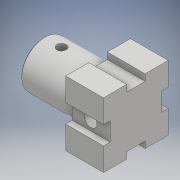
# Autodesk Inventor part: Деталь5
Saved by Autodesk Inventor 2018 (Build 220112000, 112)
## iProperties
Created: 2018-05-16
Part Number: Деталь5
Material: Типовые
Document SubType Name: Modeling
Designer: user
Density: 1 g/cm^3
Appearance: По умолчанию
Author: user
Autodesk Inventor part; units mm, degrees
ref_plane "YZ Plane" through (0, 0, 0) normal (1, 0, 0) x (0, 1, 0)
ref_plane "XZ Plane" through (0, 0, 0) normal (0, 1, 0) x (-1, 0, 0)
ref_plane "XY Plane" through (0, 0, 0) normal (0, 0, 1) x (1, 0, 0)
sketch "Эскиз1" plane through (0, 0, 0) normal (0, 0, 1) x (1, 0, 0)
  line L0 (-12.25, -21) -> (12.25, -21)
  line L1 (12.25, -21) -> (12.25, 21)
  line L2 (12.25, 21) -> (-12.25, 21)
  line L3 (-12.25, 21) -> (-12.25, -21)
  line L4 (-12.25, -21) -> (12.25, 21) construction
  line L5 (12.25, -21) -> (-12.25, 21) construction
  point P0 (0, 0)
  dimension "d0" = 24.5
  dimension "d1" = 42
  constraints: 12 end point, 2 midpoint, 2 parallel, 1 horizontal, 1 perpendicular
  measures "d0" distance of L2.end L1.end
  measures "d1" distance of L1.end L0.end
extrude "Выдавливание1" add sketch "Эскиз1" along normal mid plane 42
sketch "Эскиз2" plane through (-12.25, -21, 21) normal (-1, 0, 0) x (0, 0, 1)
  circle A0 centre (-21, 21) radius 15
  dimension "d4" = 30
  constraints: 1 centre point, 1 coincident
  measures "d4" diameter of A0
extrude "Выдавливание2" add sketch "Эскиз2" along normal blind 35
sketch "Эскиз3" plane through (-47.25, 0, 0) normal (-1, 0, 0) x (0, 0, 1)
  circle A0 centre (0, 0) radius 15 projected
  line L0 (-10, -11.1803) -> (-10, 11.1803)
  dimension "d7" = 25
  constraints: 2 end point, 2 point on circle, 1 vertical
extrude "Выдавливание3" cut sketch "Эскиз3" against normal blind 25 contours L0 A0 picked at (-11.6306, -0.5993)
chamfer "Фаска1" distance 0.5 angle 45 2 edges at (-47.25, -13.6931, 6.1237) (-47.25, 13.6931, 6.1237)
sketch "Эскиз4" plane through (-12.25, 21, 21) normal (0, 1, 0) x (1, 0, 0)
  line L0 (24.5, 42) -> (24.5, 0) projected
  line L1 (0, 15) -> (24.5, 15)
  line L2 (24.5, 15) -> (24.5, 27)
  line L3 (24.5, 27) -> (0, 27)
  line L4 (0, 27) -> (0, 15)
  line L5 (0, 15) -> (24.5, 27) construction
  line L6 (24.5, 15) -> (0, 27) construction
  point P0 (12.25, 21)
  dimension "d13" = 12
  constraints: 12 end point, 2 midpoint, 2 parallel, 1 horizontal, 1 perpendicular, 1 point on line
  measures "d13" distance of L2.end L1.end
extrude "Выдавливание4" cut sketch "Эскиз4" against normal blind 4.25
sketch "Эскиз5" plane through (-12.25, -21, 21) normal (0, -1, 0) x (1, 0, 0)
  line L0 (24.5, -42) -> (24.5, 0) projected
  line L1 (0, -15) -> (24.5, -15)
  line L2 (24.5, -15) -> (24.5, -27)
  line L3 (24.5, -27) -> (0, -27)
  line L4 (0, -27) -> (0, -15)
  line L5 (0, -15) -> (24.5, -27) construction
  line L6 (24.5, -15) -> (0, -27) construction
  point P0 (12.25, -21)
  dimension "d16" = 12
  constraints: 12 end point, 2 midpoint, 2 parallel, 1 horizontal, 1 perpendicular, 1 point on line
  measures "d16" distance of L1.end L2.end
extrude "Выдавливание5" cut sketch "Эскиз5" against normal blind 4.25
sketch "Эскиз6" plane through (0, 0, -21) normal (0, 0, -1) x (-1, 0, 0)
  line L0 (-12.25, -21) -> (-12.25, 21) projected
  line L1 (12.25, 6) -> (-12.25, 6)
  line L2 (-12.25, 6) -> (-12.25, -6)
  line L3 (-12.25, -6) -> (12.25, -6)
  line L4 (12.25, -6) -> (12.25, 6)
  line L5 (12.25, 6) -> (-12.25, -6) construction
  line L6 (-12.25, 6) -> (12.25, -6) construction
  point P0 (0, 0)
  dimension "d19" = 12
  constraints: 12 end point, 2 midpoint, 2 parallel, 1 horizontal, 1 perpendicular, 1 point on line
  measures "d19" distance of L2.end L1.end
extrude "Выдавливание6" cut sketch "Эскиз6" against normal blind 4.25
sketch "Эскиз7" plane through (0, 0, 21) normal (0, 0, 1) x (1, 0, 0)
  line L0 (-12.25, 6) -> (-12.25, -6) projected
  line L1 (12.25, 6) -> (-12.25, 6)
  line L2 (-12.25, 6) -> (-12.25, -6)
  line L3 (-12.25, -6) -> (12.25, -6)
  line L4 (12.25, -6) -> (12.25, 6)
  line L5 (12.25, 6) -> (-12.25, -6) construction
  line L6 (-12.25, 6) -> (12.25, -6) construction
  point P0 (0, 0)
  dimension "d22" = 12
  constraints: 12 end point, 2 midpoint, 2 parallel, 1 horizontal, 1 perpendicular
  measures "d22" distance of L0.end L1.end
extrude "Выдавливание7" cut sketch "Эскиз7" against normal blind 4.25
sketch "Эскиз8" plane through (-22.25, -11.1803, -10) normal (0, 0, -1) x (-1, 0, 0)
  line L0 (25, 21.6803) -> (25, 0.6803) projected
  point P0 (-22.25, 11.1803)
  point P1 (13.6, 11.1803)
  dimension "d25" = 11.4
  measures "d25" distance from line of L0 point (13.6, 11.18)
hole "Отверстие1" at (-35.85, 0, -10) direction (0, 0, 1) diameter 6 end through all
sketch "Эскиз9" plane through (-12.25, 16.75, 21) normal (0, 1, 0) x (1, 0, 0)
  line L0 (24.5, 27) -> (24.5, 15) projected
  point P0 (12.25, 21)
  point P1 (12, 21)
  dimension "d33" = 12.5
  measures "d33" distance from line of L0 point (12, 21)
hole "Отверстие2" at (-0.25, 16.75, 0) direction (0, -1, 0) diameter 8 end through all
